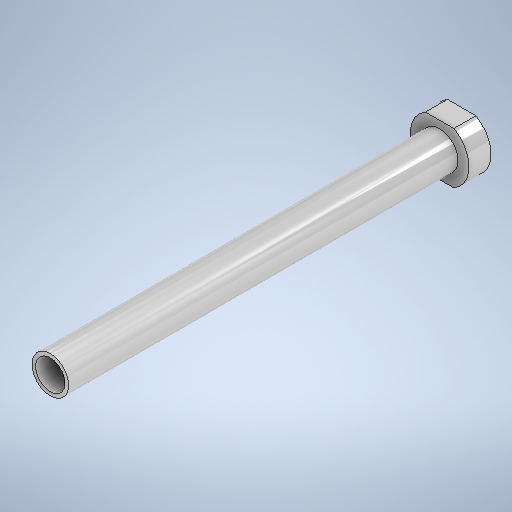
# Autodesk Inventor part: Rotation Pin
Saved by Autodesk Inventor 2025.2 (Build 292293000, 293)
## iProperties
Created: 2025-01-23
Part Number: Rotation Pin
Material: Generic
Document SubType Name: Modeling
Designer: Matt Tidd
Density: 1 g/cm^3
Appearance: Default
Mass: 1.08307 g
Surface Area: 11.0273 cm^2
Volume: 1.08307 cm^3
Author: Matt Tidd
Autodesk Inventor part; units mm, degrees
ref_plane "YZ Plane" through (0, 0, 0) normal (1, 0, 0) x (0, 1, 0)
ref_plane "XZ Plane" through (0, 0, 0) normal (0, 1, 0) x (-1, 0, 0)
ref_plane "XY Plane" through (0, 0, 0) normal (0, 0, 1) x (1, 0, 0)
sketch "Sketch1" plane through (0, 0, 0) normal (0, 0, 1) x (1, 0, 0)
  circle A0 centre (0, 0) radius 4
  line L0 (-0.0635, 3.5) -> (1.9365, 3.5)
  line L1 (-0.0635, 3.5) -> (2, 3.5) construction
  line L2 (1.9365, 3.5) -> (-1.9365, 3.5)
  line L3 (0, -3.5) -> (1.9365, -3.5)
  line L4 (1.9365, -3.5) -> (-1.9365, -3.5)
  dimension "d0" = 8
  dimension "d1" = 2
  dimension "d2" = 0
  constraints: 10 end point, 4 point on circle, 3 horizontal, 1 centre point, 1 coincident
  measures "d0" diameter of A0
  measures "d1" distance of L0.start L0.end
  measures "d2" distance between parallel lines of L0 L1
extrude "Extrusion1" add sketch "Sketch1" along normal blind 3 contours A0 L3 L4 L2 L0
sketch "Sketch2" plane through (0, 0, 3) normal (0, 0, 1) x (1, 0, 0)
  circle A0 centre (0, 0) radius 2.5
  dimension "d5" = 5
  constraints: 1 centre point, 1 coincident
  measures "d5" diameter of A0
extrude "Extrusion2" add sketch "Sketch2" along normal blind 53
sketch "Sketch3" plane through (0, 0, 56) normal (0, 0, 1) x (1, 0, 0)
  arc A0 (-1.9365, 3.5) -> (-1.9365, -3.5) centre (0, 0) ccw projected
  circle A1 centre (0, 0) radius 2
  dimension "d8" = 4
  constraints: 1 centre point, 1 coincident
  measures "d8" diameter of A1
extrude "Extrusion3" cut sketch "Sketch3" against normal blind 8
body "Solid1"
